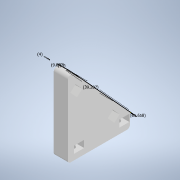
# Autodesk Inventor part: intake plate holder
Saved by Autodesk Inventor 2021 (Build 250183000, 183)
## iProperties
Created: 2021-04-01
Part Number: intake plate holder
Material: Generic
Document SubType Name: Modeling
Designer: deli
Density: 1 g/cm^3
Appearance: Default
Author: deli
Autodesk Inventor part; units mm, degrees
ref_plane "YZ Plane" through (0, 0, 0) normal (1, 0, 0) x (0, 1, 0)
ref_plane "XZ Plane" through (0, 0, 0) normal (0, 1, 0) x (-1, 0, 0)
ref_plane "XY Plane" through (0, 0, 0) normal (0, 0, 1) x (1, 0, 0)
sketch "Sketch1" plane through (0, 0, 0) normal (1, 0, 0) x (0, 1, 0)
  line L0 (28.309, -15.6604) -> (71.9614, -15.6604)
  line L1 (28.309, -55.6604) -> (28.309, -15.6604)
  line L2 (28.309, -55.6604) -> (71.9614, -15.6604)
  point P0 (0, 0)
  dimension "d2" = 42.5
  dimension "d3" = 90
  dimension "d4" = 40
  constraints: 6 end point, 1 horizontal
  measures "d2" angle of L2 L0
  measures "d3" angle of L0 L1
  measures "d4" distance of L1.start L0.start
extrude "Extrusion1" add sketch "Sketch1" along normal blind 10
sketch "Sketch2" plane through (0, 28.309, -55.6604) normal (0, -1, 0) x (1, 0, 0)
  line L0 (0, 40) -> (0, 0) projected
  line L1 (0, 0) -> (10, 0) projected
  line L2 (10, 40) -> (10, 0) projected
  line L3 (0, 40) -> (10, 40) projected
  point P0 (0, 55.6604)
extrude "Extrusion2" add sketch "Sketch2" along normal blind 10
sketch "Sketch3" plane through (0, 18.309, -55.6604) normal (0, -1, 0) x (1, 0, 0)
  arc A0 (1, 4) -> (9, 4) centre (5, 4) ccw projected
  line L0 (9, 4) -> (9, 100) projected
  arc A1 (9, 100) -> (1, 100) centre (5, 100) ccw projected
  line L1 (1, 100) -> (1, 4) projected
  circle A2 centre (5, 100) radius 2 projected
  circle A3 centre (5, 92) radius 2 projected
  circle A4 centre (5, 84) radius 2 projected
  circle A5 centre (5, 76) radius 2 projected
  circle A6 centre (5, 68) radius 2 projected
  circle A7 centre (5, 60) radius 2 projected
  circle A8 centre (5, 52) radius 2 projected
  circle A9 centre (5, 44) radius 2 projected
  circle A10 centre (5, 36) radius 2 projected
  circle A11 centre (5, 28) radius 2 projected
  circle A12 centre (5, 20) radius 2 projected
  circle A13 centre (5, 12) radius 2 projected
  circle A14 centre (5, 4) radius 2 projected
  point P0 (0, 55.6604)
extrude "Extrusion3" cut sketch "Sketch3" against normal blind 10 contours A10 | A14
sketch "Sketch4" plane through (10, 71.9614, -15.6604) normal (0, 0.6755902, -0.7372773) x (-1, 0, 0)
  line L0 (10, -59.2075) -> (10, 0) projected
  line L1 (10, 0) -> (0, 0) projected
  line L2 (0, -59.2075) -> (0, 0) projected
  line L3 (10, -59.2075) -> (0, -59.2075) projected
  circle A0 centre (5, -10) radius 2
  circle A1 centre (5, -49.2075) radius 2
  point P0 (10, -42.4755)
  dimension "d11" = 4
  dimension "d12" = 4
  dimension "d13" = 10
  dimension "d14" = 10
  constraints: 2 centre point
  measures "d11" diameter of A0
  measures "d12" diameter of A1
  measures "d13" distance from line of L1 A0.centre
  measures "d14" distance from line of L3 A1.centre
extrude "Extrusion4" cut sketch "Sketch4" against normal blind 10 contours A0 | A1
sketch "Sketch5" plane through (10, 0, 0) normal (1, 0, 0) x (0, 0, -1)
  line L0 (53.6604, 18.309) -> (53.6604, 28.309) projected
  line L1 (49.6604, 18.309) -> (49.6604, 28.309) projected
  line L2 (21.6604, 18.309) -> (21.6604, 28.309) projected
  line L3 (17.6604, 18.309) -> (17.6604, 28.309) projected
  line L4 (16.1104, 27.309) -> (23.2104, 27.309)
  line L5 (23.2104, 27.309) -> (23.2104, 22.309)
  line L6 (23.2104, 22.309) -> (16.1104, 22.309)
  line L7 (16.1104, 22.309) -> (16.1104, 27.309)
  line L8 (55.6604, 18.309) -> (15.6604, 18.309) projected
  line L9 (48.1104, 27.309) -> (55.2104, 27.309)
  line L10 (55.2104, 27.309) -> (55.2104, 22.309)
  line L11 (55.2104, 22.309) -> (48.1104, 22.309)
  line L12 (48.1104, 22.309) -> (48.1104, 27.309)
  line L13 (23.7675, 63.114) -> (16.3947, 56.3581) projected
  line L14 (21.0651, 66.0632) -> (15.6604, 61.1106) projected
  line L15 (50.2557, 34.2073) -> (42.8829, 27.4514) projected
  line L16 (47.5533, 37.1564) -> (40.1805, 30.4005) projected
  line L17 (17.0688, 64.5036) -> (21.8655, 59.2689)
  line L18 (21.8655, 59.2689) -> (18.1791, 55.891)
  line L19 (18.1791, 55.891) -> (13.3824, 61.1256)
  line L20 (13.3824, 61.1256) -> (17.0688, 64.5036)
  line L21 (55.6604, 28.309) -> (15.6604, 71.9614) projected
  line L22 (15.6604, 71.9614) -> (15.6604, 18.309) projected
  line L23 (43.557, 35.5968) -> (48.3537, 30.3621)
  line L24 (48.3537, 30.3621) -> (44.6673, 26.9842)
  line L25 (44.6673, 26.9842) -> (39.8706, 32.2188)
  line L26 (39.8706, 32.2188) -> (43.557, 35.5968)
  point P0 (0, 0)
  dimension "d17" = 7.1
  dimension "d18" = 5
  dimension "d19" = 4
  dimension "d20" = 1.55
  dimension "d21" = 4
  dimension "d22" = 7.1
  dimension "d23" = 5
  dimension "d24" = 4
  dimension "d25" = 1.55
  dimension "d28" = 7.1
  dimension "d29" = 5
  dimension "d30" = 1.55
  dimension "d31" = 4
  dimension "d33" = 7.1
  dimension "d34" = 5
  dimension "d35" = 4
  dimension "d36" = 1.55
  constraints: 32 end point, 10 parallel, 4 perpendicular, 2 horizontal
  measures "d17" distance of L5.end L6.end
  measures "d18" distance of L4.end L5.end
  measures "d19" distance between parallel lines of L2 L3
  measures "d20" distance between parallel lines of L5 L2
  measures "d21" distance between parallel lines of L8 L6
  measures "d22" distance of L10.end L11.end
  measures "d23" distance of L9.end L10.end
  measures "d24" distance between parallel lines of L8 L11
  measures "d25" distance between parallel lines of L1 L12
  measures "d28" distance of L18.end L19.end
  measures "d29" distance of L17.end L18.end
  measures "d30" distance between parallel lines of L18 L13
  measures "d31" distance between parallel lines of L21 L17
  measures "d33" distance of L24.end L25.end
  measures "d34" distance of L23.end L24.end
  measures "d35" distance between parallel lines of L21 L23
  measures "d36" distance between parallel lines of L16 L26
sketch "Sketch6" plane through (0, 71.9614, -15.6604) normal (0, 0, 1) x (1, 0, 0)
  ellipse E0 centre (5, -13.5634) end of major axis (5, -16.2761) minor radius 2 (6.7794, -14.8019) -> (3.2206, -14.8019) ccw projected
  line L0 (6.7794, -14.8019) -> (3.2206, -14.8019) projected
  line L1 (0, 0) -> (0, -53.6523) projected
  line L2 (10, -53.6523) -> (0, -53.6523) projected
  line L3 (10, 0) -> (10, -53.6523) projected
  line L4 (0, 0) -> (10, 0) projected
  point P0 (0, -71.9614)
  constraints: 1 other
extrude "Extrusion6" add sketch "Sketch6" along normal blind 4 contours L0 E0 | L4 L3 L2 L1
sketch "Sketch7" plane through (10, 28.309, -55.6604) normal (0, 0.6755902, -0.7372773) x (-1, 0, 0)
  circle A0 centre (5, 10) radius 2 projected
  circle A1 centre (5, 49.2075) radius 2 projected
  line L0 (10, 0) -> (10, 59.2075) projected
  line L1 (10, 59.2075) -> (0, 59.2075) projected
  line L2 (0, 0) -> (0, 59.2075) projected
  line L3 (10, 0) -> (0, 0) projected
  point P0 (10, 16.732)
extrude "Extrusion7" cut sketch "Sketch7" against normal blind 10 contours A1
extrude "Extrusion8" cut sketch "Sketch5" against normal blind 10 contours L11 L1 L9 L0 | L0 L9 L10 L11 | L11 L12 L9 L1 | L6 L3 L4 L2 | L2 L4 L5 L6 | L6 L7 L4 L3 | L17 L18 L19 L13 | L13 L19 L22 L14 L17 | L14 L22 L20 L17 | L19 L20 L22 | L23 L24 L25 L15 | L15 L25 L16 L23 | L16 L25 L26 L23
fillet "Fillet1" radius 2 5 edges at (5, 71.9614, -11.6604) (5, 71.9614, -15.6604) (5, 18.309, -11.6604) (5, 18.309, -55.6604) (5, 28.309, -55.6604)
sketch "Sketch8" plane through (10, 28.8825, -55.1349) normal (0, 0.6755902, -0.7372773) x (-1, 0, 0)
  line L0 (10, 0) -> (0, 0) projected
  line L1 (10, 0) -> (10, 57.5497) projected
  line L2 (0, 57.5497) -> (10, 57.5497) projected
  line L3 (0, 0) -> (0, 57.5497) projected
  circle A0 centre (5, 48.4297) radius 2 projected
  circle A1 centre (5, 9.2222) radius 2 projected
  line L4 (0, 60.3064) -> (10, 60.3064) projected
  line L5 (10, -7.3248) -> (0, -7.3248) projected
  line L6 (0, 60.3064) -> (10, 60.3064)
  line L7 (10, 60.3064) -> (10, -7.3248)
  line L8 (10, -7.3248) -> (0, -7.3248)
  line L9 (0, -7.3248) -> (0, 60.3064)
  line L10 (0, -1.3512) -> (10, -1.3512) projected
  point P0 (10, 15.9542)
  dimension "d44" = 10
  dimension "d45" = 4
  dimension "d46" = 9.8766
  dimension "d47" = 61.6575
  dimension "d48" = 39.2075
  constraints: 8 end point, 2 parallel, 1 horizontal, 1 perpendicular
  measures "d44" distance of L4.start L4.end
  measures "d45" diameter of A0
  measures "d46" distance edge to line of A0 L4
  measures "d47" distance between parallel lines of L10 L4
  measures "d48" distance of A1.centre A0.centre
equation "\"d14\" = d13"
equation "\"d20\" = -0.5 * d19 + 0.5 * d17"
equation "\"d24\" = d21"
equation "\"d25\" = d20"
equation "\"d28\" = d17"
equation "\"d29\" = d18"
equation "\"d30\" = d20"
equation "\"d31\" = d21"
equation "\"d35\" = d21"
equation "\"d36\" = d20"
body "Solid1"
